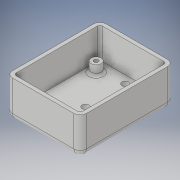
# Autodesk Inventor part: Motor_Node_box
Saved by Autodesk Inventor 2019.4 (Build 234330000, 330)
## iProperties
Created: 2019-12-12
Part Number: Motor_Node_box
Material: Generic
Document SubType Name: Modeling
Designer: Jorian Brusind
Density: 1 g/cm^3
Appearance: Default
Author: Jorian Brusind
Autodesk Inventor part; units mm, degrees
ref_plane "YZ Plane" through (0, 0, 0) normal (1, 0, 0) x (0, 1, 0)
ref_plane "XZ Plane" through (0, 0, 0) normal (0, 1, 0) x (-1, 0, 0)
sketch "Sketch1" plane through (0, 0, 0) normal (0, 1, 0) x (-1, 0, 0)
  line L0 (0, 0) -> (60, 0)
  line L1 (60, 0) -> (60, -76)
  line L2 (60, -76) -> (0, -76)
  line L3 (0, -76) -> (0, 0)
  dimension "d0" = 60
  dimension "d1" = 76
  constraints: 8 end point, 2 parallel, 1 horizontal, 1 perpendicular
  measures "d0" distance of L1.end L2.end
  measures "d1" distance of L0.end L1.end
extrude "Extrusion1" add sketch "Sketch1" along normal blind 30
sketch "Sketch2" plane through (0, 30, 0) normal (0, 1, 0) x (1, 0, 0)
  line L0 (-60, 0) -> (0, 0) projected
  line L1 (0, 0) -> (-3, 0)
  line L2 (-3, 0) -> (-3, 3)
  line L3 (-3, 3) -> (-57, 3)
  line L4 (-57, 3) -> (-57, 73)
  line L5 (-57, 73) -> (-3, 73)
  line L6 (-3, 73) -> (-3, 3)
  dimension "d4" = 3
  dimension "d5" = 3
  dimension "d6" = 54
  dimension "d7" = 70
  constraints: 12 end point, 2 parallel, 2 perpendicular, 1 horizontal, 1 point on line
  measures "d4" distance of L0.end L1.end
  measures "d5" distance of L1.end L2.end
  measures "d6" distance of L4.end L5.end
  measures "d7" distance of L3.end L4.end
extrude "Extrusion2" cut sketch "Sketch2" against normal blind 25
sketch "Sketch3" plane through (0, 5, 0) normal (0, 1, 0) x (1, 0, 0)
  line L0 (-3, 3) -> (-57, 3) projected
  line L1 (-30, 3) -> (-30, 34.3333)
  circle A0 centre (-30, 34.3333) radius 2.75
  circle A1 centre (-30, 66.6667) radius 2.75
  line L2 (-3, 73) -> (-3, 3) projected
  line L3 (-57, 73) -> (-3, 73) projected
  point P0 (0, 0)
  dimension "d10" = 31.3333
  dimension "d12" = 5.5
  dimension "d13" = 5.5
  dimension "d85" = 27
  dimension "d86" = 6.3333
  constraints: 2 centre point, 2 end point, 1 coincident, 1 midpoint, 1 vertical
  measures "d10" distance of L1.start L1.end
  measures "d12" diameter of A0
  measures "d13" diameter of A1
  measures "d85" distance from line of L2 A1.centre
  measures "d86" distance from line of L3 A1.centre
extrude "Extrusion3" cut sketch "Sketch3" against normal blind 15
sketch "Sketch4" plane through (0, 5, 0) normal (0, 1, 0) x (1, 0, 0)
  circle A0 centre (-50, 5) radius 4
  line L0 (-3, 3) -> (-57, 3) projected
  line L1 (-57, 3) -> (-57, 73) projected
  circle A1 centre (-50, 63) radius 4
  circle A2 centre (-12, 5) radius 4
  circle A3 centre (-12, 63) radius 4
  circle A4 centre (-50, 63) radius 1.75
  circle A5 centre (-50, 5) radius 1.75
  circle A6 centre (-12, 63) radius 1.75
  circle A7 centre (-12, 5) radius 1.75
  point P0 (0, 0)
  point P1 (-57, 75)
  dimension "d16" = 8
  dimension "d17" = 2
  dimension "d18" = 7
  dimension "d21" = 58
  dimension "d24" = 38
  dimension "d27" = 3.5
  dimension "d30" = 58
  dimension "d33" = 38
  constraints: 8 centre point, 2 horizontal, 2 vertical, 1 coincident, 12 other
  measures "d16" diameter of A0
  measures "d17" distance from line of L0 A0.centre
  measures "d18" distance from line of L1 A0.centre
  measures "d21" distance of A0.centre A1.centre
  measures "d24" distance of A0.centre A2.centre
  measures "d27" diameter of A4
  measures "d30" distance of A4.centre A5.centre
  measures "d33" distance of A4.centre A6.centre
extrude "Extrusion4" add sketch "Sketch4" along normal blind 8
ref_plane "Work Plane1" through (0, 0, -50) normal (0, 0, 1) x (1, 0, 0)
fillet "Fillet1" radius 5 4 edges at (0, 15, 0) (0, 15, -76) (-60, 15, -76) (-60, 15, 0)
fillet "Fillet2" radius 5 8 edges at (-1.4645, 0, -1.4645) (-30, 0, 0) (-58.5355, 0, -1.4645) (-60, 0, -38) (-58.5355, 0, -74.5355) (-30, 0, -76) (-1.4645, 0, -74.5355) (0, 0, -38)
fillet "Fillet3" radius 2 4 edges at (-50, 5, -9) (-54, 5, -63) (-12, 5, -9) (-16, 5, -63)
fillet "Fillet4" radius 2 4 edges at (-57, 17.5, -73) (-57, 17.5, -3) (-3, 17.5, -3) (-3, 17.5, -73)
body "Solid1"
